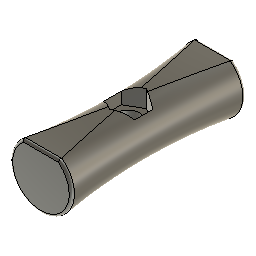
Clamptite Handle (Autodesk Fusion 360 design; units mm, degrees)
Autodesk Fusion 360 part; units mm, degrees
sketch "Sketch1" plane through (0, 0, 0) normal (0, 0, 1) x (1, 0, 0) in component "Handle"
  line L0 (6.35, 3.6662) -> (0, 7.3323)
  line L1 (0, 7.3323) -> (-6.35, 3.6662)
  line L2 (-6.35, 3.6662) -> (-6.35, -3.6662)
  line L3 (-6.35, -3.6662) -> (0, -7.3323)
  line L4 (0, -7.3323) -> (6.35, -3.6662)
  line L5 (6.35, -3.6662) -> (6.35, 3.6662)
  dimension "d1" = 6.35
  measures "d1" distance of origin L5
sketch "Sketch2" plane through (0, 0, 0) normal (0, 1, 0) x (1, 0, 0) in component "Handle"
  circle A0 centre (0, 0) radius 10
  constraint coincident A0.centre origin
ref_plane "WorkPlane1" through (0, -35, 0) normal (0, 1, 0) x (1, 0, 0) in component "Handle"
ref_plane "WorkPlane2" through (0, 35, 0) normal (0, 1, 0) x (1, 0, 0) in component "Handle"
sketch "Sketch3" plane through (0, -35, 0) normal (0, 1, 0) x (1, 0, 0) in component "Handle"
  circle A0 centre (0, 0) radius 12.5
  dimension "d4" = 25
  constraint coincident A0.centre origin
  measures "d4" diameter of A0
sketch "Sketch4" plane through (0, 35, 0) normal (0, 1, 0) x (1, 0, 0) in component "Handle"
  circle A0 centre (0, 0) radius 12.5
  dimension "d5" = 25
  constraint coincident A0.centre origin
  measures "d5" diameter of A0
loft "Loft1" add profiles "Sketch3", "Sketch2", "Sketch4" section 1 section 2 section 3 in component "Handle"
ref_plane "WorkPlane3" through (0, 0, 10) normal (0, 0, 1) x (1, 0, 0) in component "Handle"
sketch "Sketch5" plane through (0, 0, 10) normal (0, 0, 1) x (1, 0, 0) in component "Handle"
  line L0 (6.35, 3.6662) -> (0, 7.3323)
  line L1 (0, 7.3323) -> (-6.35, 3.6662)
  line L2 (-6.35, 3.6662) -> (-6.35, -3.6662)
  line L3 (-6.35, -3.6662) -> (0, -7.3323)
  line L4 (0, -7.3323) -> (6.35, -3.6662)
  line L5 (6.35, -3.6662) -> (6.35, 3.6662)
  line L6 (-14.8991, 38.6212) -> (15.1009, 38.6212)
  line L7 (15.1009, 38.6212) -> (15.1009, -36.3788)
  line L8 (15.1009, -36.3788) -> (-14.8991, -36.3788)
  line L9 (-14.8991, -36.3788) -> (-14.8991, 38.6212)
  circle A0 centre (0, 0) radius 4.5
  dimension "d7" = 6.35
  dimension "d13" = 9
  dimension "d16" = 75
  dimension "d17" = 30
  constraint coincident A0.centre origin
  constraint horizontal L6
  constraint vertical L7
  constraint horizontal L8
  constraint vertical L9
  measures "d7" distance of A0.centre L5
  measures "d13" diameter of A0
  measures "d16" distance of L6.end L7.end
  measures "d17" distance of L7.end L8.end
extrude "Extrude1" cut sketch "Sketch5" along normal mid plane 14 contours L0 L1 L2 L3 L4 L5 | A0 in component "Handle"
extrude "Extrude2" cut sketch "Sketch5" along normal blind 5 contours L6 L7 L8 L9 in component "Handle"
fillet "Fillet1" radius 1 6 edges at (5.5902, -35, -11.1803) (-11.1803, -35, 5.5902) (0, -35, 10) (0, 35, 10) (5.5902, 35, -11.1803) (-11.1803, 35, 5.5902) in component "Handle"
extrude "Extrude3" cut sketch "Sketch5" against normal blind 30 contours A0 in component "Handle"
component "Handle" placed x (1, 0, 0) y (0, 1, 0) z (0, 0, 1) at (0, 0, 0)
equation "d1 = 0.25 * 1 in"
equation "d7 = 0.25 * 1 in"
named bodies: "Handle"
